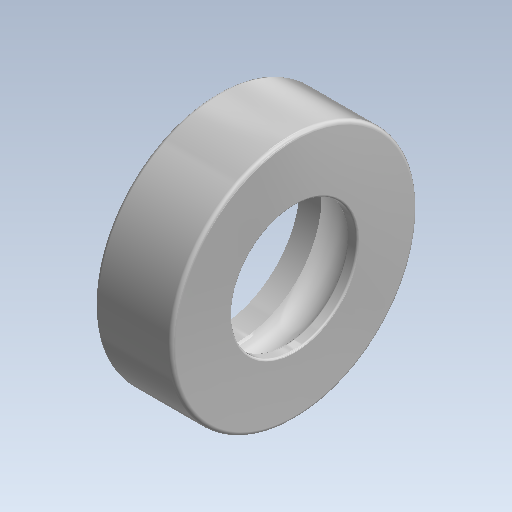
# Autodesk Inventor part: 040205DR-19-H6_or
Saved by Autodesk Inventor 2021.2 (Build 252289000, 289)
## iProperties
Part Number: 040205DR-19-H6_or
Material: アセタール樹脂、白
Catalog Web Link: www.cadenas.de
Description: DR-H or-D-Series bearings
Vendor: TOKBEARING
Document SubType Name: Modeling
Designer: partserver
Manufacturer: TOKBEARING
Mass: 8100 g
Surface Area: 10.2262 cm^2
Volume: 0.917126 cm^3
Density: 1.425 g/cm^3
Appearance: 滑らか - 白
Category: PARTsolutions
Company: TOKBEARING
PSOL_IDENT_0: {$CADENAS_DATA\23d-libs\tok_bearing\d_series_bearings\dr_h\dr_h_or.prj},177 {VTYP=3D},{NB=040205DR-1
PSOL_IDENT_1: 9-H6_or},{LINA=040205DR-19-H6_or},{NN=DR-H or},{DATE=16.12.2020 00:38:04},{GEOMDATE=19.02.2013 00:00
PSOL_IDENT_2: :00},{VERSION=},{LINEID=1520},{WBVAR=},{WBNUMERIC=}  {NB=040205DR-19-H6_or},{LINA=040205DR-19-H6_or}
PSOL_IDENT_3: ,{KT=DUMMY},{IDNR=},{CODE=040205},{PN=DR-19-H6},{D=19},{SD=6.0},{W=6.0},{W1=-},{W1X=0.000},{W2=-},{W
PSOL_IDENT_4: 2X=0.000},{LOAD=49 (5)},{TYPE=10},{QTY=2.500},{GW=8.1},{BD=3.06},{OP=35.2622},{N=5},{R=5.615},{GP=3.
PSOL_IDENT_5: 12}
NB: 040205DR-19-H6_or
NN: DR-H or
NT: D-Series bearings
NBSYN: $CODE.$PN._or
LINA: 040205DR-19-H6_or
CATALOG: TOK, Inc
CODE: 040205
PN: DR-19-H6
D: 19
SD: 6
W: 6
W1: -
W2: -
LOAD: 49 (5)
TYPE: 10
QTY: 2.500
GW: 8.1
SUPPLIER: TOKBEARING
ARTICLENO: 040205DR-19-H6_or
BOMINFO: 040205DR-19-H6_or
CREATOR: CADENAS GmbH
Title: 040205DR-19-H6_or
Author: Cadenas PARTsolutions
Comments: D-Series bearings
Autodesk Inventor part; units mm, degrees
sketch "Sketch_2" plane through (0, 0, 0) normal (0, 0, 1) x (1, 0, 0)
  line L0 (5.7, 0) -> (0.3, 0)
  line L1 (0, 9.2) -> (0, 5)
  arc A0 (0, 5) -> (0.15, 4.85) centre (0.15, 5) ccw
  line L2 (0.15, 4.85) -> (0.7071, 4.85)
  arc A1 (0.7071, 4.85) -> (0.8571, 5) centre (0.7071, 5) ccw
  line L3 (0.8571, 5) -> (0.8571, 6.38)
  line L4 (0.8571, 6.38) -> (1.675, 6.38)
  arc A2 (4.325, 6.38) -> (1.675, 6.38) centre (3, 5.615) ccw
  line L5 (4.325, 6.38) -> (6, 6.38)
  line L6 (6, 6.38) -> (6, 9.2)
  arc A3 (6, 9.2) -> (5.7, 9.5) centre (5.7, 9.2) ccw
  line L7 (5.7, 9.5) -> (0.3, 9.5)
  arc A4 (0.3, 9.5) -> (0, 9.2) centre (0.3, 9.2) ccw
  constraints: 16 end point, 10 point on circle, 5 centre point
revolve "Revolution1" add sketch "Sketch_2" angle 360 about axis through (5.7, 0, 0) along (1, 0, 0)
ref_plane "OR_Cage_XY" through (0, 0, 0) normal (1, 0, 0) x (0, 0, -1)
ref_plane "OR_Cage_YZ" through (0, 0, 0) normal (0, 0, -1) x (0, 1, 0)
ref_plane "OR_Cage_ZX" through (0, 0, 0) normal (0, 1, 0) x (1, 0, 0)
ref_plane "OR_IR_XY" through (0, 0, 0) normal (1, 0, 0) x (0, 0, -1)
ref_plane "OR_IR_YZ" through (0, 0, 0) normal (0, 0, -1) x (0, 1, 0)
ref_plane "OR_IR_ZX" through (0, 0, 0) normal (0, 1, 0) x (1, 0, 0)
ref_plane "OR_ball_1_XY" through (3, 5.615, 0) normal (1, 0, 0) x (0, 0, -1)
ref_plane "OR_ball_1_YZ" through (3, 5.615, 0) normal (0, 0, -1) x (0, 1, 0)
ref_plane "OR_ball_1_ZX" through (3, 5.615, 0) normal (0, 1, 0) x (1, 0, 0)
ref_plane "OR_ball_2_XY" through (3, 1.7351, 5.3402) normal (1, 0, 0) x (0, 0, -1)
ref_plane "OR_ball_2_YZ" through (3, 1.7351, 5.3402) normal (0, 0, -1) x (0, 1, 0)
ref_plane "OR_ball_2_ZX" through (3, 1.7351, 5.3402) normal (0, 1, 0) x (1, 0, 0)
ref_plane "OR_ball_3_XY" through (3, -4.5426, 3.3004) normal (1, 0, 0) x (0, 0, -1)
ref_plane "OR_ball_3_YZ" through (3, -4.5426, 3.3004) normal (0, 0, -1) x (0, 1, 0)
ref_plane "OR_ball_3_ZX" through (3, -4.5426, 3.3004) normal (0, 1, 0) x (1, 0, 0)
ref_plane "OR_ball_4_XY" through (3, -4.5426, -3.3004) normal (1, 0, 0) x (0, 0, -1)
ref_plane "OR_ball_4_YZ" through (3, -4.5426, -3.3004) normal (0, 0, -1) x (0, 1, 0)
ref_plane "OR_ball_4_ZX" through (3, -4.5426, -3.3004) normal (0, 1, 0) x (1, 0, 0)
ref_plane "OR_ball_5_XY" through (3, 1.7351, -5.3402) normal (1, 0, 0) x (0, 0, -1)
ref_plane "OR_ball_5_YZ" through (3, 1.7351, -5.3402) normal (0, 0, -1) x (0, 1, 0)
ref_plane "OR_ball_5_ZX" through (3, 1.7351, -5.3402) normal (0, 1, 0) x (1, 0, 0)
body "Solid1"
